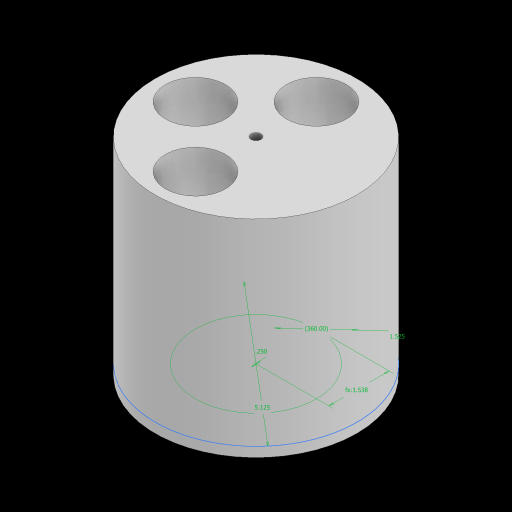
# Autodesk Inventor part: SC-1-01-Ice Core Holder
Saved by Autodesk Inventor 2023 (Build 270158000, 158)
## iProperties
Created: 2023-12-31
Part Number: SC-1-01-Ice Core Holder
Material: Generic
Document SubType Name: Modeling
Designer: annah
Density: 1 g/cm^3
Appearance: Default
Author: annah
Autodesk Inventor part; units mm, degrees
ref_plane "YZ Plane" through (0, 0, 0) normal (1, 0, 0) x (0, 1, 0)
ref_plane "XZ Plane" through (0, 0, 0) normal (0, 1, 0) x (-1, 0, 0)
sketch "Sketch2" plane through (0, 0, 0) normal (0, 1, 0) x (-1, 0, 0)
  circle A0 centre (0, 0) radius 65.0875
  circle A1 centre (0, -39.0525) radius 19.3675
  circle A2 centre (39.0525, 0) radius 19.3675
  circle A3 centre (0, 39.0525) radius 19.3675
  circle A4 centre (-39.0525, 0) radius 19.3675
  circle A5 centre (0, 0) radius 3.175
  dimension "d2" = 130.175
  dimension "d3" = 38.735
  dimension "d5" = 39.0525
  dimension "d8" = 360
  dimension "d14" = 6.35
  constraints: 6 centre point, 1 coincident, 9 other
  measures "d2" diameter of A0
  measures "d3" diameter of A1
  measures "d5" distance of point (0, 0) A1.centre
  measures "d14" diameter of A5
extrude "Extrusion1" add sketch "Sketch2" along normal blind 127 contours A0 | A4
extrude "Extrusion2" add sketch "Sketch2" against normal blind 6.35 contours A0 | A1 | A2 | A3 | A4
ref_plane "Work Plane1" through (0, 0, 65.0875) normal (0, 0, 1) x (1, 0, 0)
sketch "Sketch3" plane through (0, 0, 65.0875) normal (0, 0, 1) x (1, 0, 0)
  circle A0 centre (0, 101.6) radius 1.27
  line L0 (65.0875, 127) -> (-65.0875, 127) projected
  point P0 (0, 0)
  dimension "d16" = 2.54
  dimension "d17" = 25.4
  constraints: 1 centre point
  measures "d16" diameter of A0
  measures "d17" distance from line of L0 A0.centre
equation "\"d5\" = 0.3 * d2"
body "Solid1"
